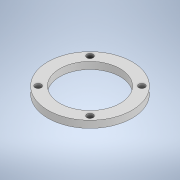
# Autodesk Inventor part: immersion_chamber_plate
Saved by Autodesk Inventor 2021 (Build 250183000, 183)
## iProperties
Created: 2021-06-16
Part Number: immersion_chamber_plate
Material: Generic
Document SubType Name: Modeling
Designer: MicroscopyInnovation
Density: 1 g/cm^3
Appearance: Default
Author: MicroscopyInnovation
Autodesk Inventor part; units mm, degrees
ref_plane "YZ Plane" through (0, 0, 0) normal (1, 0, 0) x (0, 1, 0)
ref_plane "XZ Plane" through (0, 0, 0) normal (0, 1, 0) x (-1, 0, 0)
ref_plane "XY Plane" through (0, 0, 0) normal (0, 0, 1) x (1, 0, 0)
sketch "Sketch1" plane through (0, 0, 0) normal (0, 1, 0) x (-1, 0, 0)
  circle A0 centre (0, 0) radius 21.5
  circle A1 centre (0, 0) radius 30
  dimension "d0" = 43
  dimension "d1" = 60
  constraints: 2 centre point, 2 coincident
  measures "d0" diameter of A0
  measures "d1" diameter of A1
extrude "Extrusion1" add sketch "Sketch1" along normal blind 5
sketch "Sketch2" plane through (0, 5, 0) normal (0, 1, 0) x (1, 0, 0)
  line L0 (18.5, -18.5) -> (-18.5, -18.5)
  line L1 (-18.5, -18.5) -> (-18.5, 18.5)
  line L2 (-18.5, 18.5) -> (18.5, 18.5)
  line L3 (18.5, 18.5) -> (18.5, -18.5)
  circle A0 centre (0, 0) radius 30 projected
  line L4 (18.5, -18.5) -> (-18.5, 18.5) construction
  line L5 (-18.5, -18.5) -> (18.5, 18.5) construction
  dimension "d4" = 37
  dimension "d5" = 37
  constraints: 12 end point, 2 midpoint, 2 parallel, 1 horizontal, 1 perpendicular
  measures "d4" distance of L1.end L2.end
  measures "d5" distance of L0.end L1.end
hole "Hole1" at (-18.5, 5, 18.5) at (-18.5, 5, -18.5) at (18.5, 5, -18.5) at (18.5, 5, 18.5) direction (0, -1, 0) diameter 4.496 depth 6 clearance for "Flat Head Machine Screw (82)" size "#8" standard "Ansi Unified Screw Threads"
body "Solid1"
